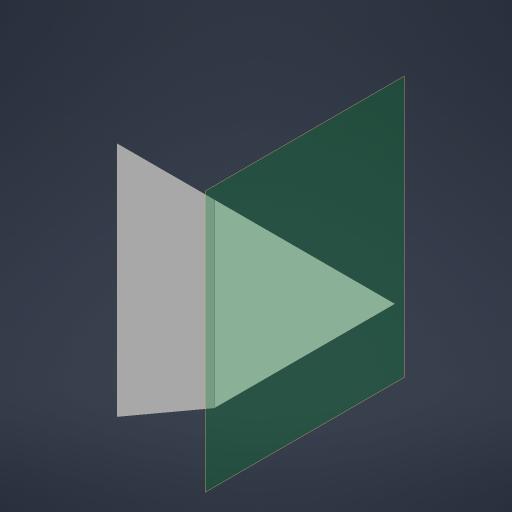
# Autodesk Inventor part: Angled_Drone_Mount
Saved by Autodesk Inventor 2023 (Build 270158000, 158)
## iProperties
Created: 2024-02-29
Part Number: Angled_Drone_Mount
Material: Generic
Document SubType Name: Modeling
Designer: kelle
Density: 1 g/cm^3
Appearance: Default
Author: kelle
Autodesk Inventor part; units mm, degrees
ref_plane "YZ Plane" through (0, 0, 0) normal (1, 0, 0) x (0, 1, 0)
ref_plane "XZ Plane" through (0, 0, 0) normal (0, 1, 0) x (-1, 0, 0)
ref_plane "XY Plane" through (0, 0, 0) normal (0, 0, 1) x (1, 0, 0)
sketch "Sketch1" plane through (0, 0, 0) normal (0, 0, 1) x (1, 0, 0)
  line L0 (25.4, -19.05) -> (-25.4, -19.05)
  line L1 (-25.4, -19.05) -> (-25.4, 19.05)
  line L2 (-25.4, 19.05) -> (25.4, 19.05)
  line L3 (25.4, 19.05) -> (25.4, -19.05)
  line L4 (25.4, -19.05) -> (-25.4, 19.05) construction
  line L5 (-25.4, -19.05) -> (25.4, 19.05) construction
  line L6 (25.4, 19.05) -> (-15.6768, -4.6657)
  line L7 (-15.6768, -4.6657) -> (-15.6768, 19.05)
  point P0 (0, 0)
  dimension "d0" = 50.8
  dimension "d1" = 38.1
  dimension "d2" = 30
  dimension "d3" = 23.7157
  dimension "d4" = 9.7232
  constraints: 16 end point, 2 midpoint, 2 parallel, 2 perpendicular, 1 horizontal, 1 point on line
  measures "d0" distance of L1.end L2.end
  measures "d1" distance of L0.end L1.end
  measures "d2" angle of L2 L6
  measures "d3" distance of L6.end L7.end
  measures "d4" distance between parallel lines of L1 L7
extrude "Extrusion1" add sketch "Sketch1" along normal blind 76.2 contours L6 L7 L2
sketch "Sketch2" plane through (-15.6768, -4.6657, 0) normal (-1, 0, 0) x (0, 0, 1)
  line L0 (0, 23.7157) -> (0, 0) projected
  line L1 (0, 0) -> (76.2, 0) projected
  line L2 (76.2, 23.7157) -> (76.2, 0) projected
  line L3 (0, 23.7157) -> (76.2, 23.7157) projected
  line L4 (0, 23.7157) -> (76.2, 23.7157)
  line L5 (76.2, 23.7157) -> (76.2, 99.9157)
  line L6 (76.2, 99.9157) -> (0, 99.9157)
  line L7 (0, 99.9157) -> (0, 23.7157)
  line L8 (0, 23.7157) -> (76.2, 99.9157)
  point P0 (0, 4.6657)
  dimension "d7" = 76.2
  dimension "d8" = 76.2
  dimension "d9" = 45
  constraints: 10 end point, 2 parallel, 1 perpendicular
  measures "d7" distance of L6.end L5.end
  measures "d8" distance of L5.end L4.end
  measures "d9" angle of L3 L8
ref_plane "Work Plane1" through (25.4, 19.05, 0) normal (-1, 0, 0) x (0, 0, 1)
extrude "Extrusion2" add sketch "Sketch2" against normal up to surface (41.0768 mm away) contours L8 L5 L3
body "Solid1"
